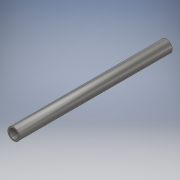
# Autodesk Inventor part: Steel Tubing
Saved by Autodesk Inventor 2017 (Build 210142000, 142)
## iProperties
Created: 2018-10-27
Part Number: Steel Tubing
Material: Stainless Steel
Document SubType Name: Modeling
Designer: Dell
Density: 8 g/cm^3
Appearance: Semi-Polished
Author: Dell
Autodesk Inventor part; units mm, degrees
ref_plane "YZ Plane" through (0, 0, 0) normal (1, 0, 0) x (0, 1, 0)
ref_plane "XZ Plane" through (0, 0, 0) normal (0, 1, 0) x (-1, 0, 0)
ref_plane "XY Plane" through (0, 0, 0) normal (0, 0, 1) x (1, 0, 0)
sketch "Sketch1" plane through (0, 0, 0) normal (0, 0, 1) x (1, 0, 0)
  circle A0 centre (0, 0) radius 4.88
  circle A1 centre (0, 0) radius 6.35
  dimension "d0" = 9.76
  dimension "d1" = 12.7
  constraints: 2 centre point, 2 coincident
  measures "d0" diameter of A0
  measures "d1" diameter of A1
extrude "Extrusion1" add sketch "Sketch1" along normal blind 160
body "Solid1"
